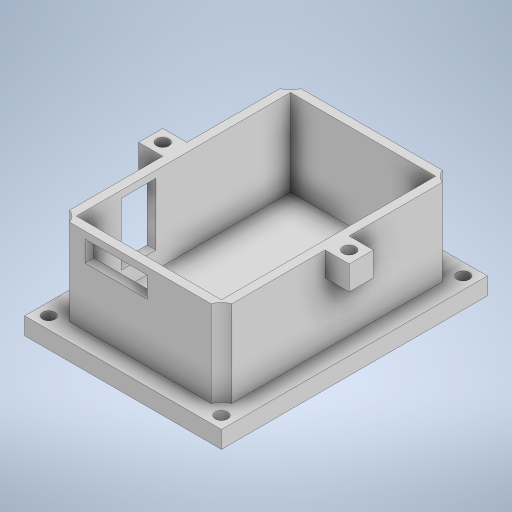
# Autodesk Inventor part: ESPBox
Saved by Autodesk Inventor 2023 (Build 270158000, 158)
## iProperties
Created: 2023-08-01
Part Number: ESPBox
Material: Generic
Document SubType Name: Modeling
Designer: campstudent
Density: 1 g/cm^3
Appearance: Default
Author: campstudent
Autodesk Inventor part; units mm, degrees
ref_plane "YZ Plane" through (0, 0, 0) normal (1, 0, 0) x (0, 1, 0)
ref_plane "XZ Plane" through (0, 0, 0) normal (0, 1, 0) x (-1, 0, 0)
ref_plane "XY Plane" through (0, 0, 0) normal (0, 0, 1) x (1, 0, 0)
sketch "Sketch1" plane through (0, 0, 0) normal (0, 1, 0) x (-1, 0, 0)
  line L0 (0, 0) -> (57, 0)
  line L1 (57, 0) -> (57, -77)
  line L2 (57, -77) -> (0, -77)
  line L3 (0, -77) -> (0, 0)
  line L4 (53.5, -3.5) -> (3.5, -3.5) construction
  line L5 (3.5, -3.5) -> (3.5, -73.5) construction
  line L6 (3.5, -73.5) -> (53.5, -73.5) construction
  line L7 (53.5, -73.5) -> (53.5, -3.5) construction
  line L8 (52, -5) -> (5, -5)
  line L9 (5, -5) -> (5, -72)
  line L10 (5, -72) -> (52, -72)
  line L11 (52, -72) -> (52, -5)
  circle A0 centre (53.5, -3.5) radius 1.8
  circle A1 centre (53.5, -73.5) radius 1.8
  circle A2 centre (3.5, -3.5) radius 1.8
  circle A3 centre (3.5, -73.5) radius 1.8
  dimension "d0" = 57
  dimension "d1" = 77
  dimension "d2" = 50
  dimension "d3" = 70
  dimension "d4" = 3.5
  dimension "d5" = 3.5
  dimension "d6" = 67
  dimension "d7" = 47
  dimension "d8" = 1.5
  dimension "d9" = 1.5
  dimension "d10" = 3.6
  dimension "d11" = 3.6
  dimension "d12" = 3.6
  dimension "d13" = 3.6
  constraints: 24 end point, 6 parallel, 4 centre point, 4 coincident, 3 horizontal, 3 perpendicular
  measures "d0" distance of L1.end L2.end
  measures "d1" distance of L0.end L1.end
  measures "d2" distance of L6.end L5.end
  measures "d3" distance of L5.end L4.end
  measures "d4" distance between parallel lines of L1 L7
  measures "d5" distance between parallel lines of L0 L4
  measures "d6" distance of L10.end L8.start
  measures "d7" distance of L9.end L10.end
  measures "d8" distance between parallel lines of L7 L11
  measures "d9" distance between parallel lines of L6 L10
  measures "d10" diameter of A0
  measures "d11" diameter of A1
  measures "d12" diameter of A2
  measures "d13" diameter of A3
extrude "Extrusion1" add sketch "Sketch1" along normal blind 5 contours L0 L1 L2 L3 | L11 L10 L9 L8
sketch "Sketch3" plane through (0, 5, 0) normal (0, 1, 0) x (1, 0, 0)
  line L0 (-52, 5) -> (-5, 5)
  line L1 (-5, 5) -> (-5, 72)
  line L2 (-5, 72) -> (-52, 72)
  line L3 (-52, 72) -> (-52, 5)
  line L4 (-57, 77) -> (-57, 0) projected
  line L5 (-57, 0) -> (0, 0) projected
  circle A0 centre (-53.5, 3.5) radius 1.8 construction
  circle A1 centre (-53.5, 3.5) radius 4.75
  circle A2 centre (-53.5, 73.5) radius 1.8 construction
  circle A3 centre (-53.5, 73.5) radius 4.75
  circle A4 centre (-3.5, 3.5) radius 1.8 construction
  circle A5 centre (-3.5, 3.5) radius 4.75
  circle A6 centre (-3.5, 73.5) radius 1.8 construction
  circle A7 centre (-3.5, 73.5) radius 4.75
  line L6 (-49.5, 7.5) -> (-7.5, 7.5)
  line L7 (-7.5, 7.5) -> (-7.5, 69.5)
  line L8 (-7.5, 69.5) -> (-49.5, 69.5)
  line L9 (-49.5, 69.5) -> (-49.5, 7.5)
  point P0 (-5, 68.9931)
  point P1 (-8.0069, 72)
  point P2 (-48.9931, 72)
  point P3 (-52, 68.9931)
  point P4 (-52, 8.0069)
  point P5 (-48.9931, 5)
  point P6 (-8.0069, 5)
  point P7 (-5, 8.0069)
  dimension "d30" = 47
  dimension "d31" = 67
  dimension "d32" = 5
  dimension "d33" = 5
  dimension "d34" = 9.5
  dimension "d35" = 9.5
  dimension "d36" = 9.5
  dimension "d37" = 9.5
  dimension "d38" = 42
  dimension "d39" = 62
  dimension "d40" = 2.5
  dimension "d41" = 2.5
  constraints: 16 end point, 4 centre point, 4 coincident, 4 parallel, 2 horizontal, 2 perpendicular
  measures "d30" distance of L2.end L1.end
  measures "d31" distance of L1.end L0.end
  measures "d32" distance between parallel lines of L4 L3
  measures "d33" distance between parallel lines of L5 L0
  measures "d34" diameter of A1
  measures "d35" diameter of A3
  measures "d36" diameter of A5
  measures "d37" diameter of A7
  measures "d38" distance of L8.end L7.end
  measures "d39" distance of L7.end L6.end
  measures "d40" distance between parallel lines of L3 L9
  measures "d41" distance between parallel lines of L0 L6
extrude "Extrusion2" add sketch "Sketch3" along normal blind 25 contours A1 L3 A3 L2 A7 L1 A5 L0
sketch "Sketch4" plane through (-48.9931, 5, -5) normal (0, 0, 1) x (1, 0, 0)
  line L0 (4.4931, 23) -> (22.4931, 23)
  line L1 (22.4931, 23) -> (22.4931, 17)
  line L2 (22.4931, 17) -> (4.4931, 17)
  line L3 (4.4931, 17) -> (4.4931, 23)
  line L4 (43.9931, 0) -> (43.9931, 25) projected
  line L5 (-8.0069, 0) -> (48.9931, 0) projected
  point P0 (48.9931, -5)
  dimension "d44" = 18
  dimension "d45" = 6
  dimension "d46" = 21.5
  dimension "d47" = 17
  constraints: 8 end point, 2 parallel, 1 horizontal, 1 perpendicular
  measures "d44" distance of L1.end L2.end
  measures "d45" distance of L0.end L1.end
  measures "d46" distance between parallel lines of L4 L1
  measures "d47" distance between parallel lines of L5 L2
extrude "Extrusion3" cut sketch "Sketch4" against normal blind 10
sketch "Sketch5" plane through (0, 30, 0) normal (0, 1, 0) x (1, 0, 0)
  line L0 (-5, 68.9931) -> (-5, 8.0069) projected
  line L1 (-5, 42) -> (2, 42)
  line L2 (2, 42) -> (2, 35)
  line L3 (2, 35) -> (-5, 35)
  line L4 (-5, 35) -> (-5, 42)
  line L5 (-8.0069, 72) -> (-48.9931, 72) projected
  line L6 (0, 77) -> (-57, 77) construction
  line L7 (-28.5, 77) -> (-28.5, 0) construction
  line L8 (-57, 0) -> (0, 0) construction
  line L9 (-5, 38.5) -> (2, 38.5) construction
  line L10 (-1.5, 42) -> (-1.5, 35) construction
  circle A0 centre (-1.5, 38.5) radius 1.8
  line L11 (-52, 42) -> (-59, 42)
  line L12 (-59, 42) -> (-59, 35)
  line L13 (-59, 35) -> (-52, 35)
  line L14 (-52, 35) -> (-52, 42)
  line L15 (-52, 38.5) -> (-59, 38.5) construction
  line L16 (-55.5, 42) -> (-55.5, 35) construction
  circle A1 centre (-55.5, 38.5) radius 1.8
  dimension "d50" = 7
  dimension "d51" = 7
  dimension "d52" = 30
  dimension "d53" = 3.6
  constraints: 26 end point, 9 symmetric about line, 7 midpoint, 2 centre point, 2 parallel, 1 horizontal, 1 perpendicular, 1 point on line, 1 other
  measures "d50" distance of L2.end L3.end
  measures "d51" distance of L1.end L2.end
  measures "d52" distance between parallel lines of L1 L5
  measures "d53" diameter of A0
extrude "Extrusion4" add sketch "Sketch5" against normal blind 7
sketch "Sketch6" plane through (-52, 5, -68.9931) normal (-1, 0, 0) x (0, 0, 1)
  line L0 (38.4931, 23) -> (48.4931, 23)
  line L1 (48.4931, 23) -> (48.4931, 5)
  line L2 (48.4931, 5) -> (38.4931, 5)
  line L3 (38.4931, 5) -> (38.4931, 23)
  line L4 (63.9931, 0) -> (63.9931, 25) projected
  line L5 (33.9931, 25) -> (60.9861, 25) projected
  line L6 (60.9861, 0) -> (0, 0) projected
  point P0 (68.9931, -5)
  dimension "d56" = 15.5
  dimension "d57" = 10
  dimension "d58" = 2
  dimension "d59" = 5
  constraints: 8 end point, 2 parallel, 1 horizontal, 1 perpendicular
  measures "d56" distance between parallel lines of L1 L4
  measures "d57" distance between parallel lines of L1 L3
  measures "d58" distance between parallel lines of L5 L0
  measures "d59" distance between parallel lines of L6 L2
extrude "Extrusion5" cut sketch "Sketch6" against normal blind 25
sketch "Sketch8" plane through (0, 5, 0) normal (0, 1, 0) x (1, 0, 0)
  line L0 (-7.5, 7.5) -> (-7.5, 69.5) projected
  line L1 (-7.5, 7.5) -> (-17.5, 7.5)
  line L2 (-17.5, 7.5) -> (-17.5, 15.5)
  line L3 (-17.5, 15.5) -> (-7.5, 15.5)
  line L4 (-7.5, 15.5) -> (-7.5, 7.5)
  line L5 (-7.5, 69.5) -> (-7.5, 7.5) projected
  line L6 (-7.5, 69.5) -> (-17.5, 69.5)
  line L7 (-17.5, 69.5) -> (-17.5, 61.5)
  line L8 (-17.5, 61.5) -> (-7.5, 61.5)
  line L9 (-7.5, 61.5) -> (-7.5, 69.5)
  point P0 (0, 0)
  dimension "d64" = 10
  dimension "d65" = 8
  dimension "d68" = 10
  dimension "d69" = 8
  constraints: 16 end point, 4 parallel, 2 horizontal, 2 perpendicular
  measures "d64" distance of L2.end L3.end
  measures "d65" distance of L1.end L2.end
  measures "d68" distance of L8.end L7.end
  measures "d69" distance of L7.end L6.end
extrude "Extrusion6" cut sketch "Sketch8" against normal blind 10
body "Solid1"
